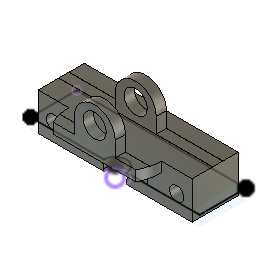
holder_1cc_hamilton v3 (Autodesk Fusion 360 design; units mm, degrees)
Autodesk Fusion 360 part; units mm, degrees
sketch "スケッチ1" plane through (0, 0, 0) normal (0, 0, 1) x (1, 0, 0)
  line L0 (-16.5, 22) -> (16.5, 22)
  line L1 (16.5, 22) -> (16.5, 0)
  line L2 (16.5, 0) -> (-16.5, 0)
  line L3 (-16.5, 0) -> (-16.5, 22)
  dimension "d7" = 22
  dimension "d8" = 33
  constraint horizontal L0
  constraint vertical L1
  constraint horizontal L2
  constraint vertical L3
  constraint coincident origin L2
  constraint midpoint origin L2
  measures "d7" distance of L0.end L1.end
  measures "d8" distance of L0.start L0.end
extrude "押し出し1" add sketch "スケッチ1" along normal blind 2
sketch "スケッチ3" plane through (0, 0, 0) normal (0, 0, -1) x (1, 0, 0)
  line L0 (16.5, 0) -> (-16.5, 0)
  line L1 (-16.5, 0) -> (-16.5, -22)
  line L2 (-16.5, -22) -> (16.5, -22)
  line L3 (16.5, -22) -> (16.5, 0)
  arc A0 (-6.3, -13) -> (6.3, -13) centre (0, -13) ccw
  line L4 (16.5, -13) -> (-16.5, -13)
  dimension "d9" = 12.6
  dimension "d10" = 9
  constraint coincident L3 L4.start
  constraint coincident L1 L4.end
  constraint perpendicular L1 L4
  constraint coincident A0.centre L4
  measures "d9" diameter of A0
  measures "d10" distance of L2 A0.centre
extrude "押し出し2" add sketch "スケッチ3" along normal blind 3.33 contours L1 L2 L3 A0 L4
sketch "スケッチ4" plane through (0, 0, -3.33) normal (0, 0, -1) x (1, 0, 0)
  line L0 (-6.3, -13) -> (-16.5, -13)
  line L1 (-16.5, -13) -> (-16.5, -22)
  line L2 (16.5, -22) -> (16.5, -13)
  line L3 (16.5, -13) -> (6.3, -13)
  arc A0 (-6.3, -13) -> (6.3, -13) centre (0, -13) ccw
  line L4 (16.5, -13) -> (16.5, -22)
  line L5 (16.5, -22) -> (-16.5, -22)
  line L6 (-16.5, -22) -> (-16.5, -13)
  arc A1 (-2.2, -13) -> (2.2, -13) centre (0, -13) ccw
  line L7 (-16.5, -13) -> (-2.2, -13)
  line L8 (2.2, -13) -> (16.5, -13)
  dimension "d88" = 4.4
  constraint horizontal L7
  constraint vertical L4
  constraint horizontal L5
  constraint vertical L6
  constraint coincident L2.start L4.end
  constraint coincident L0.end L1.start
  constraint concentric A0 A1
  constraint coincident A1.end L7
  constraint collinear L7 L8
  measures "d88" diameter of A1
extrude "押し出し3" add sketch "スケッチ4" along normal blind 2
sketch "スケッチ5" plane through (0, 0, 0) normal (0, 0, -1) x (1, 0, 0)
  line L0 (6.3, -13) -> (16.5, -13)
  line L1 (16.5, -13) -> (16.5, 0)
  line L2 (16.5, 0) -> (-16.5, 0)
  line L3 (-16.5, 0) -> (-16.5, -13)
  line L4 (-16.5, -13) -> (-6.3, -13)
  arc A0 (-6.3, -13) -> (6.3, -13) centre (0, -13) ccw
  line L5 (-3.75, 0) -> (3.75, 0)
  line L6 (3.75, 0) -> (3.75, -18)
  line L7 (3.75, -18) -> (-3.75, -18)
  line L8 (-3.75, -18) -> (-3.75, 0)
  line L9 (0, -1.75) -> (0, -22.5)
  line L10 (3.75, -7) -> (16.5, -7)
  line L11 (-3.75, -7) -> (-16.5, -7)
  dimension "d17" = 7.5
  dimension "d18" = 11
  dimension "d19" = 11
  constraint horizontal L5
  constraint vertical L6
  constraint horizontal L7
  constraint vertical L8
  constraint coincident L2 L5.start
  constraint symmetric L6 L8 L9
  constraint coincident L6 L10.start
  constraint perpendicular L6 L10
  constraint coincident L1 L10.end
  constraint coincident L8 L11.start
  constraint coincident L3 L11.end
  constraint perpendicular L3 L11
  measures "d17" distance of L5.start L5.end
  measures "d18" distance of L6.end L10.start
  measures "d19" distance of L7.end L11.start
sketch "スケッチ11" plane through (0, 22, 0) normal (0, 1, 0) x (-1, 0, 0)
  line L0 (16.5, -5.33) -> (16.5, 2)
  line L1 (16.5, 2) -> (-16.5, 2)
  line L2 (-16.5, 2) -> (-16.5, -5.33)
  line L3 (-16.5, -5.33) -> (16.5, -5.33)
  line L4 (16.5, 2) -> (-13.5, 2)
  line L5 (-13.5, 2) -> (-13.5, 12)
  line L6 (-13.5, 12) -> (16.5, 12)
  line L7 (16.5, 12) -> (16.5, 2)
  dimension "d49" = 10
  constraint horizontal L4
  constraint vertical L5
  constraint horizontal L6
  constraint vertical L7
  constraint coincident L0.end L1.start
  measures "d49" distance of L0.end L6.end
ref_plane "作業平面1" through (0, 11, -1.665) normal (0, 1, 0) x (-1, 0, 0)
sketch "スケッチ13" plane through (0, 11, -1) normal (0, 1, 0) x (1, 0, 0)
  line L0 (16.5, -10) -> (-16.5, -10)
  line L1 (-16.5, -10) -> (-16.5, -3)
  line L2 (-16.5, -3) -> (16.5, -3)
  line L3 (16.5, -3) -> (16.5, -10)
  line L4 (16.5, 4.33) -> (16.5, -3)
  line L5 (-16.5, 4.33) -> (-16.5, -3)
  circle A0 centre (0, -6.5) radius 2.25
  dimension "d53" = 7
  dimension "d54" = 4.5
  dimension "d58" = 3.5
  constraint horizontal L0
  constraint vertical L1
  constraint horizontal L2
  constraint vertical L3
  constraint collinear L3 L4
  constraint coincident L2 L1.end
  measures "d53" distance of L0.end L1.end
  measures "d54" diameter of A0
  measures "d58" distance of L2 A0.centre
extrude "押し出し11" add sketch "スケッチ13" along normal blind -2 and the other way blind -8
sketch "Sketch17" plane through (16.5, 0, 0) normal (1, 0, 0) x (0, 1, 0)
  line L0 (22, -5.33) -> (22, 2)
  line L1 (22, 2) -> (19, 2)
  line L2 (19, 2) -> (19, 9)
  line L3 (19, 9) -> (9, 9)
  line L4 (9, 9) -> (9, 2)
  line L5 (9, 2) -> (0, 2)
  line L6 (0, 2) -> (0, 0)
  line L7 (0, 0) -> (13, 0)
  line L8 (13, 0) -> (13, -5.33)
  line L9 (13, -5.33) -> (22, -5.33)
  line L10 (11, 9) -> (17, 9)
  line L11 (17, 9) -> (17, 2)
  line L12 (17, 2) -> (11, 2)
  line L13 (11, 2) -> (11, 9)
  constraint horizontal L10
  constraint vertical L11
  constraint horizontal L12
  constraint vertical L13
  constraint coincident L3 L10.start
extrude "Extrude15" cut sketch "Sketch17" against normal blind 400 contours L3 L10 L11 L12 L13
sketch "Sketch18" plane through (-16.5, 0, 0) normal (-1, 0, 0) x (0, -1, 0)
  line L0 (-11, 9) -> (-11, 2)
  line L1 (-11, 2) -> (-17, 2)
  line L2 (-17, 2) -> (-17, 9)
  line L3 (-17, 9) -> (-19, 9)
  line L4 (-19, 9) -> (-19, 2)
  line L5 (-19, 2) -> (-22, 2)
  line L6 (-22, 2) -> (-22, -5.33)
  line L7 (-22, -5.33) -> (-13, -5.33)
  line L8 (-13, -5.33) -> (-13, 0)
  line L9 (-13, 0) -> (0, 0)
  line L10 (0, 0) -> (0, 2)
  line L11 (0, 2) -> (-9, 2)
  line L12 (-9, 2) -> (-9, 9)
  line L13 (-9, 9) -> (-11, 9)
  line L14 (-9, 2) -> (0, 2)
  line L15 (0, 2) -> (0, 0)
  line L16 (0, 0) -> (-9, 0)
  line L17 (-9, 0) -> (-9, 2)
  constraint horizontal L14
  constraint vertical L15
  constraint horizontal L16
  constraint vertical L17
  constraint coincident L9.end L10.start
  constraint coincident L11.end L12.start
extrude "Extrude16" cut sketch "Sketch18" against normal blind 34 contours L9 L10 L11 L14 L15 L16 L17
sketch "Sketch19" plane through (0, 13, 0) normal (0, -1, 0) x (1, 0, 0)
  line L0 (2.2, -5.33) -> (16.5, -5.33)
  line L1 (16.5, -5.33) -> (16.5, 0)
  line L2 (16.5, 0) -> (6.3, 0)
  line L3 (6.3, 0) -> (6.3, -3.33)
  line L4 (6.3, -3.33) -> (2.2, -3.33)
  line L5 (0.6, -2) -> (16.5, -2)
  line L6 (-0.6, -2) -> (-16.5, -2)
  line L7 (2.2, -3.33) -> (2.2, -5.33)
  point P0 (12, -2)
  point P1 (-12, -2)
  constraint coincident P0 L5
  constraint coincident P1 L6
hole "Hole1" at (-12, 13, -2) at (12, 13, -2) direction (0, 1, 0) diameter 2.75 depth 5 tip angle 118
sketch "Sketch20" plane through (0, 9, 0) normal (0, -1, 0) x (1, 0, 0)
  circle A0 centre (0, 5.5) radius 2.25
  line L0 (16.5, 0) -> (16.5, 9)
  line L1 (16.5, 9) -> (-16.5, 9)
  line L2 (-16.5, 9) -> (-16.5, 0)
  line L3 (-16.5, 0) -> (16.5, 0)
  circle A1 centre (0, 5) radius 4
  line L4 (-16.5, 2, -2) -> (16.351, 2, -2)
  line L5 (16.351, 2, -2) -> (16.351, 0.0267, -2)
  line L6 (16.351, 0.0267, -2) -> (-16.5, 0.0267, -2)
  line L7 (-16.5, 0.0267, -2) -> (-16.5, 2, -2)
  line L8 (-16.5, 2.0263) -> (16.5, 2.0263)
  line L9 (16.5, 2.0263) -> (16.5, 0)
  line L10 (16.5, 0) -> (-16.5, 0)
  line L11 (-16.5, 0) -> (-16.5, 2.0263)
  line L12 (-4, 5) -> (-4, 2.0263)
  line L13 (4, 5) -> (4, 2.0263)
  point P0 (-16.5, 2)
  constraint tangent L1 A1
  constraint horizontal L8
  constraint vertical L9
  constraint horizontal L10
  constraint vertical L11
  constraint coincident L0.start L3.end
  constraint coincident L2 L8.start
  constraint coincident A1 L12.start
  constraint coincident L8 L12.end
  constraint perpendicular L8 L12
  constraint coincident A1 L13.start
  constraint coincident L8 L13.end
  constraint perpendicular L8 L13
extrude "Extrude17" cut sketch "Sketch20" against normal blind 150 contours L0 L1 A1 L8 L13 | L1 L2 A1 L8 L12
sketch "Sketch21" plane through (0, 0, -5.33) normal (0, 0, -1) x (1, 0, 0)
  line L0 (-2.2, -13) -> (-16.5, -13)
  line L1 (-16.5, -13) -> (-16.5, -22)
  line L2 (-16.5, -22) -> (16.5, -22)
  line L3 (16.5, -22) -> (16.5, -13)
  line L4 (16.5, -13) -> (2.2, -13)
  arc A0 (-2.2, -13) -> (2.2, -13) centre (0, -13) ccw
sketch "Sketch22" plane through (0, 0, 0) normal (0, 0, -1) x (1, 0, 0)
  line L0 (16.5, -9) -> (-16.5, -9)
  line L1 (-16.5, -9) -> (-16.5, -13)
  line L2 (-16.5, -13) -> (-6.3, -13)
  arc A0 (-6.3, -13) -> (6.3, -13) centre (0, -13) ccw
  line L3 (6.3, -13) -> (16.5, -13)
  line L4 (16.5, -13) -> (16.5, -9)
  circle A1 centre (0, -13) radius 9
  constraint concentric A0 A1
extrude "Extrude18" cut sketch "Sketch22" against normal blind 10 contours L0 L3 L4 A1 | L0 L1 L2 A1
move_face "OffsetFaces1" offset -1 1 faces at (16.5, 17.3333, -2.8867)
move_face "OffsetFaces2" offset -0.5 1 faces at (15.5, 17.3333, -2.8867)
move_face "OffsetFaces3" offset -1.5 1 faces at (-16.5, 17.3333, -2.8867)
move_face "OffsetFaces4" offset 1 1 faces at (5, 22, -0.4433)
move_face "OffsetFaces5" offset -1 1 faces at (5, 23, -0.4433)
fillet "Fillet1" radius 1.5 1 edges at (0, 15.2, -3.33)
